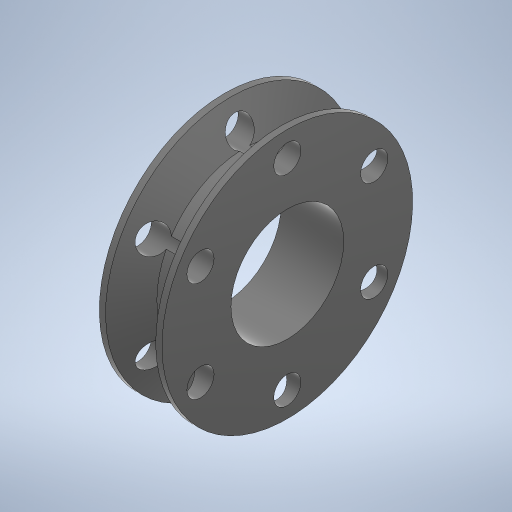
# Autodesk Inventor part: Test 2L
Saved by Autodesk Inventor 2023.2 (Build 272271000, 271)
## iProperties
Created: 2023-07-14
Part Number: Test 2L
Material: Nylon 6/6
Document SubType Name: Modeling
Designer: Nathan Cai
Mass: 5.80553 g
Surface Area: 23.5874 cm^2
Volume: 2.15019 cm^3
Density: 1.13 g/cm^3
Appearance: Smooth - Black
Author: Nathan Cai
Autodesk Inventor part; units mm, degrees
ref_plane "YZ Plane" through (0, 0, 0) normal (1, 0, 0) x (0, 1, 0)
ref_plane "XZ Plane" through (0, 0, 0) normal (0, 1, 0) x (-1, 0, 0)
ref_plane "XY Plane" through (0, 0, 0) normal (0, 0, 1) x (1, 0, 0)
sketch "Sketch1" plane through (0, 0, 0) normal (0, 0, 1) x (1, 0, 0)
  line L0 (-3.175, -2.3813) -> (3.175, -2.3813)
  line L1 (3.175, -2.3813) -> (3.175, 2.3812) construction
  line L2 (3.175, 2.3812) -> (-3.175, 2.3813)
  line L3 (-3.175, 2.3813) -> (-3.175, -2.3813) construction
  line L4 (-3.175, -2.3813) -> (3.175, 2.3812) construction
  line L5 (3.175, -2.3813) -> (-3.175, 2.3813) construction
  line L6 (0, 2.3813) -> (0, -2.3813) construction
  line L7 (-3.175, 2.3813) -> (-1.4416, -2.3813)
  line L8 (3.175, 2.3812) -> (1.4416, -2.3813)
  line L9 (-3.9688, 2.3813) -> (3.9688, 2.3813)
  line L10 (3.9688, 2.3813) -> (3.9688, -2.3813)
  line L11 (3.9688, -2.3813) -> (-3.9688, -2.3813)
  line L12 (-3.9688, -2.3813) -> (-3.9688, 2.3813)
  line L13 (-3.9688, 2.3813) -> (3.9688, -2.3813) construction
  line L14 (3.9688, 2.3813) -> (-3.9688, -2.3813) construction
  line L15 (-0.7938, 2.3813) -> (-0.7937, -2.3813) construction
  line L16 (-0.7937, -2.3813) -> (-3.9688, -2.3813)
  line L17 (-3.9688, -2.3813) -> (-3.9688, -13.4938)
  line L18 (-3.9688, -13.4938) -> (-0.7937, -13.4938)
  line L19 (-0.7937, -13.4938) -> (-0.7937, -2.3813) construction
  line L20 (3.9688, -2.3813) -> (-0.7937, -2.3813)
  line L21 (-0.7937, -2.3813) -> (-0.7937, -13.4938) construction
  line L22 (-0.7937, -13.4938) -> (3.9688, -13.4938)
  line L23 (3.9688, -13.4938) -> (3.9688, -2.3813)
  point P0 (0, 0)
  point P1 (-0.7937, -2.3813)
  dimension "d0" = 6.35
  dimension "d1" = 4.7625
  dimension "d2" = 20
  dimension "d3" = 0.7937
  dimension "d4" = 3.175
  dimension "d5" = 15.875
  constraints: 48 end point, 8 parallel, 6 midpoint, 5 perpendicular, 5 point on line, 4 horizontal, 1 symmetric about line
  measures "d0" distance of L2.end L1.end
  measures "d1" distance of L1.end L0.end
  measures "d2" angle of L6 L7
  measures "d3" distance between parallel lines of L12 L3
  measures "d4" distance between parallel lines of L12 L15
  measures "d5" distance between parallel lines of L9 L18
revolve "Revolution1" add sketch "Sketch1" angle 360 about axis through (-3.9688, -13.4938, 0) along (1, 0, 0) contours L11 L12 L9 L7 L0 | L0 L11 L23 L22 L18 L17 | L8 L9 L10 L11 L0
sketch "Sketch5" plane through (3.9688, -13.4938, 0) normal (1, 0, 0) x (0, 0, -1)
  circle A0 centre (0, 0) radius 7.1437
  circle A1 centre (0, 0) radius 15.875 construction
  circle A2 centre (0, 0) radius 12.7 construction
  line L0 (0, 0) -> (0, 12.7) construction
  circle A3 centre (0, 12.7) radius 1.7272
  circle A4 centre (-10.9985, 6.35) radius 1.7272
  circle A5 centre (-10.9985, -6.35) radius 1.7272
  circle A6 centre (0, -12.7) radius 1.7272
  circle A7 centre (10.9985, -6.35) radius 1.7272
  circle A8 centre (10.9985, 6.35) radius 1.7272
  point P0 (0, 13.4938)
  dimension "d25" = 25.4
  dimension "d24" = 14.2875
  dimension "d26" = 3.4544
  dimension "d29" = 360
  constraints: 7 centre point, 2 coincident, 2 end point, 1 concentric, 1 vertical, 1 vertical alignment, 15 other
  measures "d24" diameter of A0
  measures "d26" diameter of A3
extrude "Extrusion3" cut sketch "Sketch5" against normal through all
body "Solid1"
